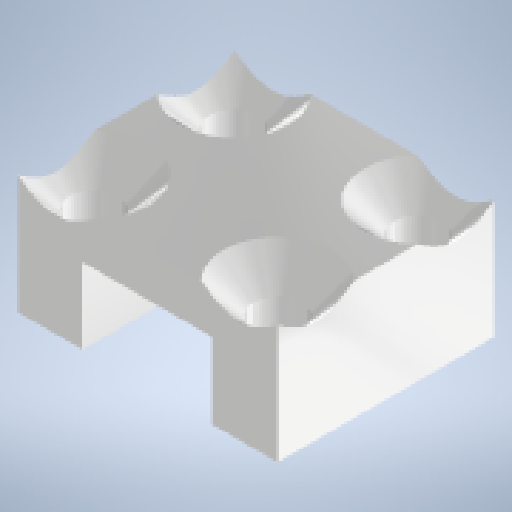
# Autodesk Inventor part: Sliderhalter
Saved by Autodesk Inventor 2025 (Build 290162010, 162A)
## iProperties
Created: 2024-11-26
Part Number: Sliderhalter
Material: PC/ABS-Kunststoff, 3DDruck, PLA
Document SubType Name: Modeling
Designer: Admin
Density: 1.1 g/cm^3
Appearance: Glatt - Weiß(2)
Author: Admin
Autodesk Inventor part; units mm, degrees
ref_plane "YZ Plane" through (0, 0, 0) normal (1, 0, 0) x (0, 1, 0)
ref_plane "XZ Plane" through (0, 0, 0) normal (0, 1, 0) x (-1, 0, 0)
ref_plane "XY Plane" through (0, 0, 0) normal (0, 0, 1) x (1, 0, 0)
sketch "Skizze1" plane through (0, 0, 0) normal (0, 0, 1) x (1, 0, 0)
  line L0 (49.8801, -4.4448) -> (46.8801, -4.4448)
  line L1 (46.8801, -4.4448) -> (46.8801, -14.4448)
  line L2 (46.8801, -14.4448) -> (49.8801, -14.4448)
  line L3 (49.8801, -14.4448) -> (49.8801, -4.4448)
  line L4 (46.8801, -14.4448) -> (40.8801, -14.4448)
  line L5 (40.8801, -14.4448) -> (40.8801, -4.4448)
  line L6 (40.8801, -4.4448) -> (46.8801, -4.4448)
  line L7 (46.8801, -4.4448) -> (46.8801, -14.4448)
  line L8 (40.8801, -14.4448) -> (37.8801, -14.4448)
  line L9 (37.8801, -14.4448) -> (37.8801, -4.4448)
  line L10 (37.8801, -4.4448) -> (40.8801, -4.4448)
  line L11 (40.8801, -4.4448) -> (40.8801, -14.4448)
  point P0 (0, 0)
  dimension "d0" = 3
  dimension "d1" = 10
  dimension "d2" = 6
  dimension "d3" = 3
  constraints: 24 end point, 6 parallel, 3 horizontal, 3 perpendicular, 2 point on line
  measures "d0" distance of L2.end L1.end
  measures "d1" distance of L1.end L0.end
  measures "d2" distance of L5.end L6.end
  measures "d3" distance of L9.end L10.end
extrude "Extrusion1" add sketch "Skizze1" along normal blind 3.5 contours L3 L2 L1 L0 | L5 L8 L9 L10
sketch "Skizze2" plane through (0, 0, 3.5) normal (0, 0, 1) x (1, 0, 0)
  line L0 (49.8801, -14.4448) -> (37.8801, -14.4448)
  line L1 (49.8801, -4.4448) -> (37.8801, -4.4448)
  line L2 (37.8801, -4.4448) -> (37.8801, -14.4448) projected
  line L3 (49.8801, -14.4448) -> (49.8801, -4.4448) projected
  point P0 (0, 0)
  constraints: 4 end point, 1 parallel
extrude "Extrusion2" add sketch "Skizze2" along normal blind 2
sketch "Skizze3" plane through (0, 0, 5.5) normal (0, 0, 1) x (1, 0, 0)
  line L0 (37.8801, -4.4448) -> (37.8801, -14.4448) projected
  line L1 (39.6301, -6.1948) -> (37.8801, -6.1948) construction
  line L2 (39.6301, -6.1948) -> (41.3801, -6.1948) construction
  line L3 (39.6301, -6.1948) -> (39.6301, -4.4448) construction
  line L4 (48.1301, -6.1948) -> (49.8801, -6.1948) construction
  line L5 (49.8801, -4.4448) -> (37.8801, -4.4448) construction
  line L6 (39.6301, -12.6948) -> (39.6301, -14.4448) construction
  line L7 (49.8801, -14.4448) -> (49.8801, -4.4448) projected
  line L8 (48.1301, -12.6948) -> (48.1301, -14.4448) construction
  line L9 (48.1301, -12.6948) -> (49.8801, -12.6948) construction
  line L10 (49.8801, -14.4448) -> (37.8801, -14.4448)
  line L11 (37.8801, -14.4448) -> (49.8801, -14.4448) projected
  point P0 (0, 0)
  dimension "d24" = 1.75
  constraints: 16 end point, 10 point on line, 6 equal length, 3 perpendicular, 2 collinear, 2 horizontal, 1 vertical
  measures "d24" distance of L1.start L1.end
hole "Bohrung1" at (39.6301, -6.1948, 5.5) at (39.6301, -12.6948, 5.5) at (48.1301, -6.1948, 5.5) at (48.1301, -12.6948, 5.5) direction (0, 0, -1) diameter 2.2 end through all countersink diameter 5 countersink angle 90
